Autodesk Inventor part; units mm, degrees
(part 2 of 2)
sketch "Эскиз2" plane through (0, 0, 1.5) normal (0, 0, 1) x (1, 0, 0)
  circle A0 centre (6.1, 396.5) radius 1.625 projected
  line L0 (280, 81) -> (280, 325) projected
  line L1 (280, 325) -> (380, 325) projected
  line L2 (380, 325) -> (380, 406) projected
  line L3 (380, 406) -> (0, 406) projected
  line L4 (0, 406) -> (0, 0) projected
  line L5 (0, 0) -> (380, 0) projected
  line L6 (380, 0) -> (380, 81) projected
  line L7 (380, 81) -> (280, 81) projected
  circle A1 centre (103.5763, 396.5) radius 1.625 projected
  circle A2 centre (276.4236, 396.5) radius 1.625 projected
  circle A3 centre (189.9999, 396.5) radius 1.625 projected
  circle A4 centre (373.8998, 396.5) radius 1.625 projected
  circle A5 centre (6.1, 396.5) radius 1.625 projected
  circle A6 centre (103.5763, 9.5) radius 1.625 projected
  circle A7 centre (373.8998, 9.5) radius 1.625 projected
  circle A8 centre (276.4236, 9.5) radius 1.625 projected
  circle A9 centre (189.9999, 9.5) radius 1.625 projected
  circle A10 centre (6.1, 9.5) radius 1.625 projected
  line L8 (0, 203) -> (395.2875, 203)
  line L9 (6.1, 332.0468) -> (6.1, 396.5)
  arc A11 (25.7748, 382.773) -> (24.6115, 379.1461) centre (25.7748, 380.773) ccw
  arc A12 (19.2632, 378.0528) -> (16.1, 376.4258) centre (18.1, 376.4258) ccw
  line L10 (16.1, 347.773) -> (16.1, 376.4258)
  arc A13 (16.1, 347.773) -> (18.1, 345.773) centre (18.1, 347.773) ccw
  line L11 (25.7748, 382.773) -> (65.85, 382.773)
  line L12 (59.3385, 349.3999) -> (19.2632, 378.0528)
  line L13 (58.1752, 345.773) -> (18.1, 345.773)
  line L14 (67.85, 345.773) -> (16.1, 382.773)
  line L15 (64.6868, 352.2342) -> (24.6115, 379.1461)
  arc A14 (67.85, 380.773) -> (65.85, 382.773) centre (65.85, 380.773) ccw
  line L16 (67.85, 380.773) -> (67.85, 353.8612)
  arc A15 (58.1752, 345.773) -> (59.3385, 349.3999) centre (58.1752, 347.773) ccw
  arc A16 (64.6868, 352.2342) -> (67.85, 353.8612) centre (65.85, 353.8612) ccw
  line L17 (113.5763, 373.5) -> (113.5763, 425.0371)
  line L18 (199.9999, 373.5) -> (199.9999, 468.6033)
  line L19 (286.4236, 373.5) -> (286.4236, 463.5998)
  line L20 (6.1, 396.5) -> (337.0883, 396.5)
  arc A17 (155.6515, 345.773) -> (156.8147, 349.3999) centre (155.6515, 347.773) ccw
  line L21 (113.5763, 347.773) -> (113.5763, 376.4258)
  arc A18 (113.5763, 347.773) -> (115.5763, 345.773) centre (115.5763, 347.773) ccw
  line L22 (155.6515, 345.773) -> (115.5763, 345.773)
  line L23 (123.251, 382.773) -> (163.3263, 382.773)
  line L24 (156.8147, 349.3999) -> (116.7395, 378.0528)
  arc A19 (123.251, 382.773) -> (122.0878, 379.1461) centre (123.251, 380.773) ccw
  arc A20 (116.7395, 378.0528) -> (113.5763, 376.4258) centre (115.5763, 376.4258) ccw
  arc A21 (162.1631, 352.2342) -> (165.3263, 353.8612) centre (163.3263, 353.8612) ccw
  line L25 (165.3263, 380.773) -> (165.3263, 353.8612)
  arc A22 (165.3263, 380.773) -> (163.3263, 382.773) centre (163.3263, 380.773) ccw
  line L26 (162.1631, 352.2342) -> (122.0878, 379.1461)
  line L27 (165.3263, 345.773) -> (113.5763, 382.773)
  arc A23 (242.0752, 345.773) -> (243.2384, 349.3999) centre (242.0752, 347.773) ccw
  line L28 (199.9999, 347.773) -> (199.9999, 376.4258)
  arc A24 (199.9999, 347.773) -> (201.9999, 345.773) centre (201.9999, 347.773) ccw
  line L29 (242.0752, 345.773) -> (201.9999, 345.773)
  line L30 (209.6747, 382.773) -> (249.7499, 382.773)
  line L31 (243.2384, 349.3999) -> (203.1631, 378.0528)
  arc A25 (209.6747, 382.773) -> (208.5115, 379.1461) centre (209.6747, 380.773) ccw
  arc A26 (203.1631, 378.0528) -> (199.9999, 376.4258) centre (201.9999, 376.4258) ccw
  arc A27 (248.5867, 352.2342) -> (251.7499, 353.8612) centre (249.7499, 353.8612) ccw
  line L32 (251.7499, 380.773) -> (251.7499, 353.8612)
  arc A28 (251.7499, 380.773) -> (249.7499, 382.773) centre (249.7499, 380.773) ccw
  line L33 (248.5867, 352.2342) -> (208.5115, 379.1461)
  line L34 (251.7499, 345.773) -> (199.9999, 382.773)
  arc A29 (328.4988, 345.773) -> (329.662, 349.3999) centre (328.4988, 347.773) ccw
  line L35 (286.4236, 347.773) -> (286.4236, 376.4258)
  arc A30 (286.4236, 347.773) -> (288.4236, 345.773) centre (288.4236, 347.773) ccw
  line L36 (328.4988, 345.773) -> (288.4236, 345.773)
  line L37 (296.0983, 382.773) -> (336.1736, 382.773)
  line L38 (329.662, 349.3999) -> (289.5868, 378.0528)
  arc A31 (296.0983, 382.773) -> (294.9351, 379.1461) centre (296.0983, 380.773) ccw
  arc A32 (289.5868, 378.0528) -> (286.4236, 376.4258) centre (288.4236, 376.4258) ccw
  arc A33 (335.0103, 352.2342) -> (338.1736, 353.8612) centre (336.1736, 353.8612) ccw
  line L39 (338.1736, 380.773) -> (338.1736, 353.8612)
  arc A34 (338.1736, 380.773) -> (336.1736, 382.773) centre (336.1736, 380.773) ccw
  line L40 (335.0103, 352.2342) -> (294.9351, 379.1461)
  line L41 (338.1736, 345.773) -> (286.4236, 382.773)
  circle A35 centre (6.1, 9.5) radius 1.625
  line L42 (280, 81) -> (380, 81)
  line L43 (380, 81) -> (380, 0)
  line L44 (380, 0) -> (0, 0)
  circle A36 centre (373.8998, 73.9532) radius 1.625
  circle A37 centre (189.9999, 73.9532) radius 1.625
  circle A38 centre (6.1, 73.9532) radius 1.625
  circle A39 centre (103.5763, 9.5) radius 1.625
  circle A40 centre (276.4236, 9.5) radius 1.625
  circle A41 centre (189.9999, 9.5) radius 1.625
  circle A42 centre (373.8998, 9.5) radius 1.625
  circle A43 centre (6.1, 9.5) radius 1.625
  circle A44 centre (103.5763, 73.9532) radius 1.625
  circle A45 centre (276.4236, 73.9532) radius 1.625
  line L45 (6.1, 73.9532) -> (6.1, 9.5)
  arc A46 (59.3385, 56.6001) -> (58.1752, 60.227) centre (58.1752, 58.227) ccw
  line L46 (16.1, 58.227) -> (16.1, 29.5742)
  arc A47 (18.1, 60.227) -> (16.1, 58.227) centre (18.1, 58.227) ccw
  line L47 (58.1752, 60.227) -> (18.1, 60.227)
  line L48 (25.7748, 23.227) -> (65.85, 23.227)
  line L49 (59.3385, 56.6001) -> (19.2632, 27.9472)
  arc A48 (24.6115, 26.8539) -> (25.7748, 23.227) centre (25.7748, 25.227) ccw
  arc A49 (16.1, 29.5742) -> (19.2632, 27.9472) centre (18.1, 29.5742) ccw
  arc A50 (67.85, 52.1388) -> (64.6868, 53.7658) centre (65.85, 52.1388) ccw
  line L50 (67.85, 25.227) -> (67.85, 52.1388)
  arc A51 (65.85, 23.227) -> (67.85, 25.227) centre (65.85, 25.227) ccw
  line L51 (64.6868, 53.7658) -> (24.6115, 26.8539)
  line L52 (67.85, 60.227) -> (16.1, 23.227)
  line L53 (113.5763, 32.5) -> (113.5763, -19.0371)
  line L54 (199.9999, 32.5) -> (199.9999, -62.6033)
  line L55 (286.4236, 32.5) -> (286.4236, -57.5998)
  line L56 (6.1, 9.5) -> (337.0883, 9.5)
  arc A52 (122.0878, 26.8539) -> (123.251, 23.227) centre (123.251, 25.227) ccw
  arc A53 (113.5763, 29.5742) -> (116.7395, 27.9472) centre (115.5763, 29.5742) ccw
  arc A54 (163.3263, 23.227) -> (165.3263, 25.227) centre (163.3263, 25.227) ccw
  arc A55 (156.8147, 56.6001) -> (155.6515, 60.227) centre (155.6515, 58.227) ccw
  line L57 (123.251, 23.227) -> (163.3263, 23.227)
  line L58 (165.3263, 25.227) -> (165.3263, 52.1388)
  line L59 (162.1631, 53.7658) -> (122.0878, 26.8539)
  arc A56 (165.3263, 52.1388) -> (162.1631, 53.7658) centre (163.3263, 52.1388) ccw
  line L60 (156.8147, 56.6001) -> (116.7395, 27.9472)
  line L61 (165.3263, 60.227) -> (113.5763, 23.227)
  line L62 (155.6515, 60.227) -> (115.5763, 60.227)
  arc A57 (115.5763, 60.227) -> (113.5763, 58.227) centre (115.5763, 58.227) ccw
  line L63 (113.5763, 58.227) -> (113.5763, 29.5742)
  arc A58 (208.5115, 26.8539) -> (209.6747, 23.227) centre (209.6747, 25.227) ccw
  arc A59 (199.9999, 29.5742) -> (203.1631, 27.9472) centre (201.9999, 29.5742) ccw
  arc A60 (249.7499, 23.227) -> (251.7499, 25.227) centre (249.7499, 25.227) ccw
  arc A61 (243.2384, 56.6001) -> (242.0752, 60.227) centre (242.0752, 58.227) ccw
  line L64 (209.6747, 23.227) -> (249.7499, 23.227)
  line L65 (251.7499, 25.227) -> (251.7499, 52.1388)
  line L66 (248.5867, 53.7658) -> (208.5115, 26.8539)
  arc A62 (251.7499, 52.1388) -> (248.5867, 53.7658) centre (249.7499, 52.1388) ccw
  line L67 (243.2384, 56.6001) -> (203.1631, 27.9472)
  line L68 (251.7499, 60.227) -> (199.9999, 23.227)
  line L69 (242.0752, 60.227) -> (201.9999, 60.227)
  arc A63 (201.9999, 60.227) -> (199.9999, 58.227) centre (201.9999, 58.227) ccw
  line L70 (199.9999, 58.227) -> (199.9999, 29.5742)
  arc A64 (294.9351, 26.8539) -> (296.0983, 23.227) centre (296.0983, 25.227) ccw
  arc A65 (286.4236, 29.5742) -> (289.5868, 27.9472) centre (288.4236, 29.5742) ccw
  arc A66 (336.1736, 23.227) -> (338.1736, 25.227) centre (336.1736, 25.227) ccw
  arc A67 (329.662, 56.6001) -> (328.4988, 60.227) centre (328.4988, 58.227) ccw
  line L71 (296.0983, 23.227) -> (336.1736, 23.227)
  line L72 (338.1736, 25.227) -> (338.1736, 52.1388)
  line L73 (335.0103, 53.7658) -> (294.9351, 26.8539)
  arc A68 (338.1736, 52.1388) -> (335.0103, 53.7658) centre (336.1736, 52.1388) ccw
  line L74 (329.662, 56.6001) -> (289.5868, 27.9472)
  line L75 (338.1736, 60.227) -> (286.4236, 23.227)
  line L76 (328.4988, 60.227) -> (288.4236, 60.227)
  arc A69 (288.4236, 60.227) -> (286.4236, 58.227) centre (288.4236, 58.227) ccw
  line L77 (286.4236, 58.227) -> (286.4236, 29.5742)
  point P0 (16.1, 382.773)
  point P1 (16.1, 396.5)
  point P2 (113.5763, 396.5)
  point P3 (199.9999, 396.5)
  point P4 (286.4236, 396.5)
  point P5 (16.1, 23.227)
  point P6 (16.1, 9.5)
  point P7 (113.5763, 9.5)
  point P8 (199.9999, 9.5)
  point P9 (286.4236, 9.5)
  dimension "d91" = 37
  dimension "d92" = 51.75
  dimension "d93" = 47.75
  dimension "d94" = 4.3472
  dimension "d95" = 33
  dimension "d96" = 2
  dimension "d97" = 2
  dimension "d98" = 2
  dimension "d99" = 2
  dimension "d100" = 2
  dimension "d101" = 2
  dimension "d102" = 28.6528
  dimension "d103" = 2
  dimension "d105" = 37
  dimension "d106" = 51.75
  dimension "d107" = 47.75
  dimension "d108" = 4.3472
  dimension "d109" = 33
  dimension "d110" = 2
  dimension "d111" = 2
  dimension "d112" = 2
  dimension "d113" = 2
  dimension "d114" = 2
  dimension "d115" = 2
  dimension "d116" = 28.6528
  dimension "d117" = 2
  dimension "d118" = 37
  dimension "d119" = 51.75
  dimension "d120" = 47.75
  dimension "d121" = 4.3472
  dimension "d122" = 33
  dimension "d123" = 2
  dimension "d124" = 2
  dimension "d125" = 2
  dimension "d126" = 2
  dimension "d127" = 2
  dimension "d128" = 2
  dimension "d129" = 28.6528
  dimension "d130" = 2
  dimension "d131" = 37
  dimension "d132" = 51.75
  dimension "d133" = 47.75
  dimension "d134" = 4.3472
  dimension "d135" = 33
  dimension "d136" = 2
  dimension "d137" = 2
  dimension "d138" = 2
  dimension "d139" = 2
  dimension "d140" = 2
  dimension "d141" = 2
  dimension "d142" = 28.6528
  dimension "d143" = 2
  constraints: 140 end point, 102 symmetric about line, 96 point on circle, 59 centre point, 46 point on line, 3 vertical, 2 horizontal, 1 midpoint, 1 parallel, 30 other
  measures "d91" distance between parallel lines of L13 L11
  measures "d92" distance between parallel lines of L16 L10
  measures "d93" horizontal distance of A14.centre A13.centre
  measures "d94" vertical distance of A11.centre A12.centre
  measures "d95" vertical distance of A15.centre A11.centre
  measures "d96" radius of A11
  measures "d97" radius of A12
  measures "d98" radius of A13
  measures "d99" radius of A15
  measures "d100" radius of A14
  measures "d101" radius of A16
  measures "d102" distance of L10.start L10.end
  measures "d103" distance from line of A12.centre L10
  measures "d105" distance between parallel lines of L22 L23
  measures "d106" distance between parallel lines of L25 L21
  measures "d107" horizontal distance of A22.centre A18.centre
  measures "d108" vertical distance of A19.centre A20.centre
  measures "d109" vertical distance of A17.centre A19.centre
  measures "d110" radius of A19
  measures "d111" radius of A20
  measures "d112" radius of A18
  measures "d113" radius of A17
  measures "d114" radius of A22
  measures "d115" radius of A21
  measures "d116" distance of L21.start L21.end
  measures "d117" distance from line of A20.centre L21
  measures "d118" distance between parallel lines of L29 L30
  measures "d119" distance between parallel lines of L32 L28
  measures "d120" horizontal distance of A28.centre A24.centre
  measures "d121" vertical distance of A25.centre A26.centre
  measures "d122" vertical distance of A23.centre A25.centre
  measures "d123" radius of A25
  measures "d124" radius of A26
  measures "d125" radius of A24
  measures "d126" radius of A23
  measures "d127" radius of A28
  measures "d128" radius of A27
  measures "d129" distance of L28.start L28.end
  measures "d130" distance from line of A26.centre L28
  measures "d131" distance between parallel lines of L36 L37
  measures "d132" distance between parallel lines of L39 L35
  measures "d133" horizontal distance of A34.centre A30.centre
  measures "d134" vertical distance of A31.centre A32.centre
  measures "d135" vertical distance of A29.centre A31.centre
  measures "d136" radius of A31
  measures "d137" radius of A32
  measures "d138" radius of A30
  measures "d139" radius of A29
  measures "d140" radius of A34
  measures "d141" radius of A33
  measures "d142" distance of L35.start L35.end
  measures "d143" distance from line of A32.centre L35
extrude "Выдавливание2" cut sketch "Эскиз2" against normal blind 1.5 contours L11 A14 L16 A16 L15 A11 | L12 A15 L13 A13 L10 A12 | L17 A20 L24 A17 L22 A18 L21 | L18 A26 L31 A23 L29 A24 L28 | L19 A32 L38 A29 L36 A30 L35 | L23 A22 L25 A21 L26 A19 | L30 A28 L32 A27 L33 A25 | L37 A34 L39 A33 L40 A31 | A36 | A37 | A38 | A44 | A45 | L49 A49 L46 A47 L47 A46 | A48 L51 A50 L50 A51 L48 | L63 A57 L62 A55 L60 A53 L53 | L70 A63 L69 A61 L67 A59 L54 | L77 A69 L76 A67 L74 A65 L55 | L59 A56 L58 A54 L57 A52 | L66 A62 L65 A60 L64 A58 | L73 A68 L72 A66 L71 A64
sketch "Эскиз4" plane through (0, 0, 1.5) normal (0, 0, 1) x (1, 0, 0)
  line L0 (391.3464, 129.9271) -> (391.3464, 259.9271) projected
  line L1 (199.3064, 259.9271) -> (391.3464, 259.9271) projected
  line L2 (199.3064, 129.9271) -> (199.3064, 259.9271) projected
  line L3 (391.3464, 129.9271) -> (199.3064, 129.9271) projected
  circle A0 centre (6.1, 9.5) radius 1.625 projected
  circle A1 centre (189.9999, 9.5) radius 1.625 projected
  circle A2 centre (276.4236, 9.5) radius 1.625 projected
  circle A3 centre (373.8998, 9.5) radius 1.625 projected
  circle A4 centre (103.5763, 9.5) radius 1.625 projected
  circle A5 centre (6.1, 396.5) radius 1.625 projected
  circle A6 centre (373.8998, 396.5) radius 1.625 projected
  circle A7 centre (189.9999, 396.5) radius 1.625 projected
  circle A8 centre (276.4236, 396.5) radius 1.625 projected
  circle A9 centre (103.5763, 396.5) radius 1.625 projected
  line L4 (0, 406) -> (0, 0) projected
  line L5 (0, 0) -> (380, 0) projected
  line L6 (380, 0) -> (380, 81) projected
  line L7 (380, 81) -> (280, 81) projected
  line L8 (280, 81) -> (280, 325) projected
  line L9 (280, 325) -> (380, 325) projected
  line L10 (380, 325) -> (380, 406) projected
  line L11 (380, 406) -> (0, 406) projected
  line L12 (235, 259.9271) -> (235, 129.9271)
  line L13 (240.6723, 129.9271) -> (240.6723, 259.9271)
  line L14 (280, 81) -> (235, 81)
  line L15 (235, 81) -> (235, 325)
  line L16 (235, 325) -> (280, 325)
  line L17 (280, 325) -> (280, 81)
  point P0 (280, 129.9271)
  point P1 (280, 259.9271)
  point P2 (280, 325)
  dimension "d72" = 45
  constraints: 12 end point, 4 point on line, 3 perpendicular, 2 parallel, 1 horizontal
  measures "d72" distance between parallel lines of L8 L12
extrude "Выдавливание4" cut sketch "Эскиз4" against normal blind 10 contours L8 L14 L15 L3 | L3 L13 L1 L8 | L1 L15 L16 L8 | L3 L12 L1 L13
sketch "Эскиз5" plane through (0, 0, 1.5) normal (0, 0, 1) x (1, 0, 0)
  line L0 (235, 325) -> (380, 325) projected
  line L1 (380, 325) -> (380, 406) projected
  line L2 (380, 406) -> (0, 406) projected
  line L3 (0, 406) -> (0, 0) projected
  line L4 (0, 0) -> (380, 0) projected
  line L5 (380, 0) -> (380, 81) projected
  line L6 (380, 81) -> (235, 81) projected
  line L7 (235, 81) -> (235, 325) projected
  circle A0 centre (103.5763, 396.5) radius 1.625 projected
  circle A1 centre (276.4236, 396.5) radius 1.625 projected
  circle A2 centre (189.9999, 396.5) radius 1.625 projected
  circle A3 centre (373.8998, 396.5) radius 1.625 projected
  circle A4 centre (6.1, 396.5) radius 1.625 projected
  circle A5 centre (103.5763, 9.5) radius 1.625 projected
  circle A6 centre (373.8998, 9.5) radius 1.625 projected
  circle A7 centre (276.4236, 9.5) radius 1.625 projected
  circle A8 centre (189.9999, 9.5) radius 1.625 projected
  circle A9 centre (6.1, 9.5) radius 1.625 projected
  line L8 (0, 406) -> (0, 0) projected
  line L9 (0, 203) -> (170, 203)
  circle A10 centre (170, 203) radius 4
  dimension "d75" = 170
  dimension "d76" = 8
  constraints: 2 end point, 1 centre point, 1 coincident, 1 horizontal, 1 midpoint
  measures "d75" distance of L9.start L9.end
  measures "d76" diameter of A10
extrude "Выдавливание5" cut sketch "Эскиз5" against normal blind 10 contours A10
sketch "Эскиз6" plane through (0, 0, 1.5) normal (0, 0, 1) x (1, 0, 0)
  circle A0 centre (170, 203) radius 4 projected
  line L0 (170, 203) -> (270, 203)
  line L1 (235, 325) -> (380, 325) projected
  line L2 (235, 81) -> (235, 325) projected
  line L3 (380, 81) -> (235, 81) projected
  line L4 (270, 325) -> (270, 81)
  point P0 (0, 0)
  dimension "d79" = 100
  dimension "d82" = 0
  constraints: 4 end point, 2 point on line, 1 horizontal, 1 perpendicular
  measures "d79" distance of L0.start L0.end
  measures "d82" distance from line of L4 L0.end
extrude "Выдавливание6" add sketch "Эскиз6" against normal up to surface (1.5 mm away) contours L2 L1 L4 L0 | L0 L4 L3 L2
sketch "Эскиз7" plane through (0, 0, 0) normal (0, 0, -1) x (-1, 0, 0)
  arc A0 (-163.05, 168.1192) -> (-167.05, 168.1192) centre (-165.05, 169.15) ccw projected
  arc A1 (-167.05, 218.1808) -> (-163.05, 218.1808) centre (-165.05, 217.15) ccw projected
  arc A2 (-176.95, 218.1808) -> (-172.95, 218.1808) centre (-174.95, 217.15) ccw projected
  arc A3 (-172.95, 168.1192) -> (-176.95, 168.1192) centre (-174.95, 169.15) ccw projected
  circle A4 centre (-174.95, 169.15) radius 2.25
  circle A5 centre (-165.05, 169.15) radius 2.25
  line L0 (-160, 173.7) -> (-160, 212) projected
  line L1 (-180, 212) -> (-180, 173.7) projected
  line L2 (-179, 213) -> (-173.14, 213) projected
  line L3 (-166.86, 213) -> (-161, 213) projected
  line L4 (-160, 213) -> (-180, 213)
  line L5 (-180, 213) -> (-180, 172.7)
  line L6 (-180, 172.7) -> (-160, 172.7)
  line L7 (-160, 172.7) -> (-160, 213)
  line L8 (-181, 213.85) -> (-159, 213.85)
  line L9 (-159, 213.85) -> (-159, 171.85)
  line L10 (-159, 171.85) -> (-181, 171.85)
  line L11 (-181, 171.85) -> (-181, 213.85)
  line L12 (-181, 213.85) -> (-159, 171.85) construction
  line L13 (-159, 213.85) -> (-181, 171.85) construction
  circle A6 centre (-165.05, 217.15) radius 2.25
  circle A7 centre (-174.95, 217.15) radius 2.25
  circle A8 centre (-170, 203) radius 4 projected
  circle A9 centre (-170, 203) radius 30.3
  circle A10 centre (-170, 233.3) radius 2.1
  circle A11 centre (-196.2406, 187.85) radius 2.1
  circle A12 centre (-143.7594, 187.85) radius 2.1
  point P0 (0, 0)
  point P1 (-170, 192.85)
  point P2 (-176.95, 218.1808)
  point P3 (-163.05, 218.1808)
  point P4 (-167.05, 168.1192)
  point P5 (-176.95, 168.1192)
  dimension "d144" = 20
  dimension "d145" = 40.3
  dimension "d146" = 22
  dimension "d147" = 42
  dimension "d157" = 4.2
  dimension "d160" = 360
  constraints: 20 end point, 7 centre point, 5 coincident, 4 concentric, 4 parallel, 3 horizontal, 2 midpoint, 2 perpendicular, 1 vertical alignment, 9 other
  measures "d144" distance of L6.end L5.end
  measures "d145" distance of L5.end L4.end
  measures "d146" distance of L9.end L10.end
  measures "d147" distance of L8.end L9.end
  measures "d157" diameter of A10
extrude "Выдавливание7" cut sketch "Эскиз7" against normal blind 22 contours A5 A0 | A6 A1 | A7 A2 | A4 A3 | L7 L6 A9 L0 | L0 A9 L9 L10 L11 L1 L5 L6 L7 | A9 L1 L5 L4 L2 L3 L7 L0 | L0 L7 L4 L3 L2 L5 L1 A9 L11 L8 L9 | L6 L5 L1 A9 | A12 A9 | A9 A12 | A11 A9 | A9 A11 | A10 A9 | A9 A10 | A8
ref_plane "РабПлоскость1" through (270, 203, 1.5) normal (0, -1, 0) x (1, 0, 0)
mirror "Зеркальное отражение1" about plane through (270, 203, 1.5) normal (0, -1, 0) of "Выдавливание2"
